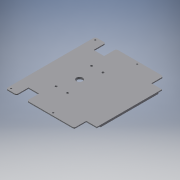
# Autodesk Inventor part: vrch1
Saved by Autodesk Inventor 2016 (Build 200138000, 138)
## iProperties
Created: 2015-11-06
Part Number: vrch1
Material: Generic
Document SubType Name: Modeling
Designer: Jufo
Density: 1 g/cm^3
Appearance: Default
Author: Jufo
Autodesk Inventor part; units mm, degrees
ref_plane "YZ Plane" through (0, 0, 0) normal (1, 0, 0) x (0, 1, 0)
ref_plane "XZ Plane" through (0, 0, 0) normal (0, 1, 0) x (-1, 0, 0)
ref_plane "XY Plane" through (0, 0, 0) normal (0, 0, 1) x (1, 0, 0)
sketch "Sketch1" plane through (0, 0, 0) normal (0, 1, 0) x (-1, 0, 0)
  line L0 (-66.8277, -81.8282) -> (-43.7605, -81.8282)
  line L1 (-43.7605, -81.8282) -> (-43.7605, -108.8282)
  line L2 (-43.7605, -108.8282) -> (-43.7605, -81.8282)
  line L3 (-43.7605, -108.8282) -> (42.2395, -108.8282)
  line L4 (42.2395, -108.8282) -> (-43.7605, -108.8282)
  line L5 (42.2395, -108.8282) -> (42.2395, -81.8282)
  line L6 (42.2395, -81.8282) -> (66.2395, -81.8282)
  line L7 (66.2395, -81.8282) -> (66.2395, -108.8282)
  line L8 (66.2395, -108.8282) -> (82.1723, -108.8282)
  line L9 (82.1723, -108.8282) -> (82.1723, 57.1718)
  line L10 (82.1723, 57.1718) -> (66.2395, 57.1718)
  line L11 (66.2395, 57.1718) -> (82.1723, 57.1718)
  line L12 (66.2395, 30.1718) -> (42.2395, 30.1718)
  line L13 (42.2395, 30.1718) -> (42.2395, 57.1718)
  line L14 (42.2395, 30.1718) -> (42.2395, 57.1718)
  line L15 (42.2395, 57.1718) -> (-43.7605, 57.1718)
  line L16 (-43.7605, 30.1718) -> (-66.8277, 30.1718)
  line L17 (-66.8277, 30.1718) -> (-43.7605, 30.1718)
  line L18 (-66.8277, 30.1718) -> (-66.8277, -81.8282)
  circle A0 centre (79.2395, -105.8282) radius 1.5
  circle A1 centre (79.2395, -105.8282) radius 1.5
  circle A2 centre (79.2395, 54.1718) radius 1.5
  circle A3 centre (79.2395, 54.1718) radius 1.5
  circle A4 centre (-0.7605, 54.1718) radius 1.5
  circle A5 centre (-0.7605, 54.1718) radius 1.5
  circle A6 centre (-0.7605, -105.8282) radius 1.5
  line L19 (-43.7605, 57.1718) -> (-43.7605, 30.1718)
  line L20 (82.1723, 57.1718) -> (81.1723, 57.1718)
  line L21 (82.1723, 57.1718) -> (82.1723, 56.1718)
  line L22 (66.2395, 57.1718) -> (66.2395, 30.1718)
  line L23 (67.2395, 30.1718) -> (67.2395, 29.1718)
  line L24 (67.2395, 29.1718) -> (42.2395, 29.1718)
  line L25 (42.2395, 57.1718) -> (41.2395, 57.1718)
  line L26 (41.2395, 29.1718) -> (42.2395, 29.1718)
  line L27 (42.2395, 57.1718) -> (42.2395, 56.1718)
  line L28 (-43.7605, 57.1718) -> (-42.7605, 57.1718)
  line L29 (-66.8277, 30.1718) -> (-67.7605, 30.1718)
  line L30 (67.2395, 56.1718) -> (67.2395, 29.1718)
  line L31 (67.2395, 56.1718) -> (81.1723, 56.1718)
  line L32 (81.1723, 56.1718) -> (81.1723, -107.8282)
  line L33 (41.2395, 56.1718) -> (-42.7605, 56.1718)
  line L34 (-42.7605, 56.1718) -> (-42.7605, 29.1718)
  line L35 (41.2395, 56.1718) -> (41.2395, 29.1718)
  line L36 (-65.8277, 29.1718) -> (-65.8277, -80.8282)
  line L37 (-42.7605, 29.1718) -> (-65.8277, 29.1718)
  line L38 (67.2395, -80.8282) -> (42.2395, -80.8282)
  line L39 (41.2395, -80.8282) -> (42.2395, -80.8282)
  line L40 (67.2395, -107.8282) -> (67.2395, -80.8282)
  line L41 (67.2395, -107.8282) -> (81.1723, -107.8282)
  line L42 (41.2395, -107.8282) -> (-42.7605, -107.8282)
  line L43 (-42.7605, -107.8282) -> (-42.7605, -80.8282)
  line L44 (41.2395, -107.8282) -> (41.2395, -80.8282)
  line L45 (-42.7605, -80.8282) -> (-65.8277, -80.8282)
  point P0 (0, 0)
  point P1 (0, 0)
  point P2 (-65.7605, 30.1718)
  dimension "d0" = 1
  dimension "d1" = 1
  dimension "d2" = 1
  dimension "d3" = 1
  dimension "d4" = 1
  dimension "d5" = 1
  dimension "d6" = 1
  dimension "d97" = 1
  dimension "d99" = 84
  dimension "d100" = 25
  dimension "d101" = 27
  dimension "d102" = 1
  dimension "d103" = 147
  dimension "d104" = 1
  constraints: 92 end point, 10 point on line, 7 centre point, 7 perpendicular, 5 collinear, 3 coincident, 3 parallel, 2 horizontal, 2 vertical
  measures "d0" distance of L12.start L23.start
  measures "d1" distance of L9.end L20.end
  measures "d2" distance of L9.end L21.end
  measures "d3" distance of L23.start L23.end
  measures "d4" distance of L13.end L25.end
  measures "d5" distance of L13.end L27.end
  measures "d6" distance of L15.end L28.end
  measures "d97" distance between parallel lines of L18 L36
  measures "d99" distance of L33.start L33.end
  measures "d100" distance of L23.end L24.end
  measures "d101" distance of L30.start L23.end
  measures "d102" distance between parallel lines of L34 L19
  measures "d103" distance between parallel lines of L36 L32
  measures "d104" distance between parallel lines of L32 L9
extrude "Extrusion1" add sketch "Sketch1" along normal blind 2 contours L30 L31 L32 L41 L40 L38 L39 L44 L42 L43 L45 L36 L37 L34 L33 L35 L26 L24 L23
sketch "Sketch4" plane through (0, 2, 0) normal (0, 1, 0) x (1, 0, 0)
  line L0 (65.7605, -36.1718) -> (45.7605, -36.1718)
  line L1 (45.7605, -36.1718) -> (45.7605, -59.1718)
  line L2 (45.7605, -59.1718) -> (-44.2395, -59.1718)
  line L3 (-44.2395, -59.1718) -> (-44.2395, -36.1718)
  line L4 (-44.2395, -59.1718) -> (-44.2395, -36.1718)
  line L5 (-44.2395, -36.1718) -> (-64.2395, -36.1718)
  line L6 (-64.2395, -36.1718) -> (-64.2395, -59.1718)
  line L7 (-64.2395, -59.1718) -> (-84.1723, -59.1718)
  line L8 (-84.1723, -59.1718) -> (-84.1723, 110.8282)
  line L9 (-84.1723, -59.1718) -> (-84.1723, 110.8282)
  line L10 (-84.1723, 110.8282) -> (-64.2395, 110.8282)
  line L11 (-64.2395, 110.8282) -> (-64.2395, 87.8282)
  line L12 (-64.2395, 87.8282) -> (-44.2395, 87.8282)
  line L13 (-44.2395, 87.8282) -> (-44.2395, 110.8282)
  line L14 (-44.2395, 87.8282) -> (-44.2395, 110.8282)
  line L15 (-44.2395, 110.8282) -> (45.7605, 110.8282)
  line L16 (45.7605, 110.8282) -> (45.7605, 87.8282)
  line L17 (45.7605, 87.8282) -> (65.7605, 87.8282)
  line L18 (65.8277, 80.8282) -> (42.7605, 80.8282) projected
  line L19 (-41.2395, -56.1718) -> (42.7605, -56.1718) projected
  line L20 (-41.2395, 80.8282) -> (-67.2395, 80.8282) projected
  line L21 (-81.1723, 107.8282) -> (-81.1723, -56.1718) projected
  line L22 (42.7605, -56.1718) -> (42.7605, -29.1718) projected
  line L23 (65.8277, -29.1718) -> (65.8277, 80.8282) projected
  line L24 (-67.2395, 80.8282) -> (-67.2395, 107.8282) projected
  line L25 (-67.2395, 107.8282) -> (-81.1723, 107.8282) projected
  line L26 (-67.2395, -56.1718) -> (-67.2395, -29.1718) projected
  line L27 (-67.2395, -29.1718) -> (-41.2395, -29.1718) projected
  line L28 (42.7605, -29.1718) -> (65.8277, -29.1718) projected
  line L29 (65.7605, 87.8282) -> (65.8277, 87.8282)
  line L30 (65.8277, 87.8282) -> (65.8277, -36.1718)
  line L31 (65.7605, -36.1718) -> (65.8277, -36.1718)
  point P0 (-0.4583, 54.4093)
  point P1 (-0.4583, 54.4093)
  point P2 (65.7605, -59.1718)
  point P3 (65.7605, 110.8282)
  point P4 (67.7605, 110.8282)
  point P5 (67.7605, -59.1718)
  dimension "d40" = 2
  dimension "d53" = 3
  dimension "d54" = 3
  dimension "d55" = 3
  dimension "d56" = 3
  dimension "d57" = 3
  dimension "d58" = 3
  dimension "d59" = 7
  dimension "d60" = 3
  dimension "d61" = 3
  dimension "d62" = 3
  dimension "d63" = 7
  constraints: 42 end point, 7 point on line, 1 horizontal, 1 perpendicular
  measures "d40" distance of point (65.76, 110.828) point (67.76, 110.828)
  measures "d53" horizontal distance of L20.start L13.start
  measures "d54" distance from line of L24 L12.start
  measures "d55" distance between parallel lines of L25 L10
  measures "d56" distance between parallel lines of L9 L21
  measures "d57" horizontal distance of L8.start L21.end
  measures "d58" distance from line of L26 L6.end
  measures "d59" distance between parallel lines of L27 L5
  measures "d60" horizontal distance of L2.end L19.start
  measures "d61" horizontal distance of L2.end L19.start
  measures "d62" horizontal distance of L1.end L19.end
  measures "d63" distance between parallel lines of L28 L0
extrude "Extrusion2" add sketch "Sketch4" along normal blind 2
sketch "Sketch5" plane through (0, 0, 0) normal (0, -1, 0) x (1, 0, 0)
  circle A0 centre (0.7605, 54.1718) radius 1.5 projected
  circle A1 centre (0.7605, 54.1718) radius 1.5
  circle A2 centre (0.7605, -105.8282) radius 1.5 projected
  circle A3 centre (0.7605, -105.8282) radius 1.5
  circle A4 centre (-79.2395, 54.1718) radius 1.5 projected
  circle A5 centre (-79.2395, 54.1718) radius 1.5
  circle A6 centre (-79.2395, -105.8282) radius 1.5 projected
  circle A7 centre (-79.2395, -105.8282) radius 1.5
  point P0 (0, 0)
  constraints: 4 centre point, 4 coincident
extrude "Extrusion3" cut sketch "Sketch5" against normal blind 4
sketch "Sketch8" plane through (0, 4, 0) normal (0, 1, 0) x (1, 0, 0)
  circle A0 centre (-29.0841, 25.8282) radius 6
  line L0 (-29.0841, 25.8282) -> (-43.0841, 25.8282)
  line L1 (-43.0841, 25.8282) -> (-43.0841, 21.3282)
  circle A1 centre (-43.0841, 21.3282) radius 2
  circle A2 centre (-43.0841, 27.2184) radius 2
  line L2 (-29.0841, 25.8282) -> (4.9159, 25.8282)
  line L3 (4.9159, 25.8282) -> (4.9159, 18.2184)
  circle A3 centre (4.9159, 18.2184) radius 2
  circle A4 centre (4.9159, 27.2184) radius 2
  circle A5 centre (-29.0841, 25.8282) radius 35.46
  line L4 (-19.0841, 59.849) -> (-39.0841, 59.849)
  circle A6 centre (-18.1693, 59.5666) radius 2
  line L5 (-29.0841, -9.6318) -> (-29.0841, 40.8935)
  circle A7 centre (-39.9988, 59.5666) radius 2
  circle A8 centre (-18.1693, -7.9102) radius 2
  circle A9 centre (-39.9988, -7.9102) radius 2
  line L6 (-44.2395, -59.1718) -> (45.7605, -59.1718) projected
  line L7 (-84.1723, 110.8282) -> (-84.1723, -59.1718) projected
  point P0 (0, 0)
  point P1 (0, 0)
  dimension "d71" = 12
  dimension "d72" = 14
  dimension "d73" = 4.5
  dimension "d74" = 4
  dimension "d75" = 34
  dimension "d76" = 4
  dimension "d77" = 70.92
  dimension "d78" = 20
  dimension "d79" = 4
  dimension "d80" = 85
  constraints: 12 end point, 10 centre point, 4 point on circle, 3 coincident, 3 symmetric about line, 2 vertical, 1 horizontal, 1 perpendicular, 3 other
  measures "d71" diameter of A0
  measures "d72" distance of L0.start L0.end
  measures "d73" distance of L0.end L1.end
  measures "d74" diameter of A1
  measures "d75" distance of L0.start L2.end
  measures "d76" diameter of A3
  measures "d77" diameter of A5
  measures "d78" distance of L4.start L4.end
  measures "d79" diameter of A6
  measures "d80" distance between parallel lines of L6 L2
extrude "Extrusion4" cut sketch "Sketch8" against normal blind 5 contours L2 L5 A0 | A0 L5 L2 | L5 L0 A0 | A0 L0 L5 | A9 A5 | A5 A9 | A8 A5 | A5 A8 | A6 L4 A5 | A5 A6 | L4 A6 A5 | A7 A5 | A5 L4 A7 | L4 A5 A7
sketch "Sketch9" plane through (0, 0, 0) normal (0, -1, 0) x (1, 0, 0)
  arc A0 (7.1961, -19.635) -> (7.1961, -22.635) centre (5.5191, -21.135) ccw
  circle A1 centre (5.5191, -21.135) radius 2.25
  arc A2 (7.1961, -29.135) -> (7.1961, -32.135) centre (5.5191, -30.635) ccw
  circle A3 centre (5.5191, -30.635) radius 2.25
  arc A4 (-45.158, -22.635) -> (-45.158, -19.635) centre (-43.4809, -21.135) ccw
  circle A5 centre (-43.4809, -21.135) radius 2.25
  arc A6 (-45.158, -32.135) -> (-45.158, -29.135) centre (-43.4809, -30.635) ccw
  circle A7 centre (-43.4809, -30.635) radius 2.25
  circle A8 centre (-29.0898, -25.885) radius 6.4
  circle A9 centre (-29.0898, -25.885) radius 5.3776
  circle A10 centre (5.5191, -21.135) radius 3
  circle A11 centre (5.5191, -30.635) radius 3
  circle A12 centre (5.5191, -21.135) radius 1.5
  circle A13 centre (5.5191, -30.635) radius 1.5
  circle A14 centre (-43.4809, -21.135) radius 1.5
  circle A15 centre (-43.4809, -21.135) radius 3
  circle A16 centre (-43.4809, -30.635) radius 1.5
  circle A17 centre (-43.4809, -30.635) radius 3
  point P0 (0, 0)
  point P1 (0, 0)
  point P2 (-18.9809, -25.885)
  dimension "d84" = 6
  dimension "d85" = 6
  dimension "d86" = 3
  dimension "d87" = 3
  dimension "d88" = 3
  dimension "d89" = 6
  dimension "d90" = 3
  dimension "d91" = 6
  constraints: 18 centre point, 13 coincident, 8 point on circle
  measures "d84" diameter of A10
  measures "d85" diameter of A11
  measures "d86" diameter of A12
  measures "d87" diameter of A13
  measures "d88" diameter of A14
  measures "d89" diameter of A15
  measures "d90" diameter of A16
  measures "d91" diameter of A17
extrude "Extrusion5" add sketch "Sketch9" along normal blind 11 contours A1 A0 | A3 A2 | A5 A4 | A7 A6 | A10 | A11 | A15 | A17
fillet "Fillet1" radius 3 8 edges at (-84.1723, 3, 59.1718) (-64.2395, 3, 59.1718) (-44.2395, 3, 59.1718) (45.7605, 3, 59.1718) (-84.1723, 3, -110.8282) (-64.2395, 3, -110.8282) (-44.2395, 3, -110.8282) (45.7605, 3, -110.8282)
body "Solid1"
